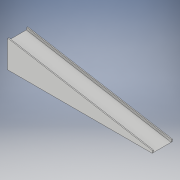
# Autodesk Inventor part: rampe-rendmonnaie
Saved by Autodesk Inventor 2019 (Build 230136000, 136)
## iProperties
Created: 2018-12-30
Part Number: rampe-rendmonnaie
Material: Générique
Document SubType Name: Modeling
Designer: pouey
Density: 1 g/cm^3
Appearance: Par défaut
Author: pouey
Autodesk Inventor part; units mm, degrees
ref_plane "YZ Plane" through (0, 0, 0) normal (1, 0, 0) x (0, 1, 0)
ref_plane "XZ Plane" through (0, 0, 0) normal (0, 1, 0) x (-1, 0, 0)
ref_plane "XY Plane" through (0, 0, 0) normal (0, 0, 1) x (1, 0, 0)
sketch "Esquisse2" plane through (0, 0, 0) normal (0, 0, 1) x (1, 0, 0)
  line L0 (0, 0) -> (0, 50)
  line L1 (0, 50) -> (290, 0)
  line L2 (290, 0) -> (0, 0)
  dimension "d0" = 290
  dimension "d1" = 50
  constraints: 6 end point, 1 perpendicular, 1 vertical
  measures "d0" distance of L1.end L0.start
  measures "d1" distance of L0.start L0.end
extrude "Extrusion1" add sketch "Esquisse2" along normal blind 40
sketch "Esquisse3" plane through (0, 50, 40) normal (0.1699069, 0.9854601, 0) x (0.9854601, -0.1699069, 0)
  line L0 (0, 40) -> (0, 0) projected
  line L1 (0, 2) -> (294.2788, 2)
  line L2 (294.2788, 40) -> (294.2788, 0) projected
  line L3 (0, 38) -> (294.2788, 38)
  line L4 (0, 40) -> (294.2788, 40) projected
  line L5 (294.2788, 0) -> (0, 0) projected
  point P0 (8.4953, 40)
  dimension "d5" = 2
  dimension "d6" = 2
  constraints: 4 end point, 4 point on line, 1 horizontal, 1 perpendicular
  measures "d5" distance between parallel lines of L4 L3
  measures "d6" distance between parallel lines of L5 L1
extrude "Extrusion2" add sketch "Esquisse3" along normal blind 5 contours L4 L2 L3 L0 | L1 L2 L5 L0
